Autodesk Fusion 360 part; units mm, degrees
note: some values were not read from the file. Set by a fixed rule: the direction of a hole.
(part 8 of 10)
  arc A350 (11.303, 28.321) -> (11.049, 28.575) centre (11.049, 28.321) ccw
  arc A351 (9.017, 28.321) -> (9.271, 28.575) centre (9.271, 28.321) cw
  line L6255 (11.049, 22.225) -> (9.271, 22.225)
  line L6256 (9.017, 22.479) -> (9.017, 22.86)
  line L6257 (9.144, 22.987) -> (9.017, 22.86)
  line L6258 (11.303, 22.479) -> (11.303, 22.86)
  line L6259 (11.176, 22.987) -> (11.303, 22.86)
  line L6260 (9.144, 27.813) -> (9.017, 27.94)
  line L6261 (9.144, 27.813) -> (9.144, 22.987)
  line L6262 (11.176, 27.813) -> (11.303, 27.94)
  line L6263 (11.176, 27.813) -> (11.176, 22.987)
  line L6264 (9.017, 28.321) -> (9.017, 27.94)
  line L6265 (11.303, 28.321) -> (11.303, 27.94)
  line L6266 (11.049, 28.575) -> (9.271, 28.575)
  line L6267 (9.8552, 28.575) -> (10.4648, 28.575)
  line L6268 (10.4648, 29.4386) -> (9.8552, 29.4386)
  line L6269 (9.8552, 29.4386) -> (9.8552, 28.575)
  line L6270 (10.4648, 28.575) -> (10.4648, 29.4386)
  line L6271 (9.8552, 22.225) -> (9.8552, 21.3614)
  line L6272 (9.8552, 21.3614) -> (10.4648, 21.3614)
  line L6273 (10.4648, 21.3614) -> (10.4648, 22.225)
  line L6274 (10.4648, 22.225) -> (9.8552, 22.225)
  arc A352 (21.971, 22.225) -> (21.717, 22.479) centre (21.971, 22.479) cw
  arc A353 (23.749, 22.225) -> (24.003, 22.479) centre (23.749, 22.479) ccw
  arc A354 (24.003, 28.321) -> (23.749, 28.575) centre (23.749, 28.321) ccw
  arc A355 (21.717, 28.321) -> (21.971, 28.575) centre (21.971, 28.321) cw
  line L6275 (23.749, 22.225) -> (21.971, 22.225)
  line L6276 (21.717, 22.479) -> (21.717, 22.86)
  line L6277 (21.844, 22.987) -> (21.717, 22.86)
  line L6278 (24.003, 22.479) -> (24.003, 22.86)
  line L6279 (23.876, 22.987) -> (24.003, 22.86)
  line L6280 (21.844, 27.813) -> (21.717, 27.94)
  line L6281 (21.844, 27.813) -> (21.844, 22.987)
  line L6282 (23.876, 27.813) -> (24.003, 27.94)
  line L6283 (23.876, 27.813) -> (23.876, 22.987)
  line L6284 (21.717, 28.321) -> (21.717, 27.94)
  line L6285 (24.003, 28.321) -> (24.003, 27.94)
  line L6286 (23.749, 28.575) -> (21.971, 28.575)
  line L6287 (22.5552, 28.575) -> (23.1648, 28.575)
  line L6288 (22.5552, 29.4386) -> (22.5552, 28.575)
  line L6289 (23.1648, 29.4386) -> (22.5552, 29.4386)
  line L6290 (23.1648, 28.575) -> (23.1648, 29.4386)
  line L6291 (22.5552, 21.3614) -> (23.1648, 21.3614)
  line L6292 (23.1648, 22.225) -> (22.5552, 22.225)
  line L6293 (23.1648, 21.3614) -> (23.1648, 22.225)
  line L6294 (22.5552, 22.225) -> (22.5552, 21.3614)
  arc A356 (34.671, 22.225) -> (34.417, 22.479) centre (34.671, 22.479) cw
  arc A357 (36.449, 22.225) -> (36.703, 22.479) centre (36.449, 22.479) ccw
  arc A358 (36.703, 28.321) -> (36.449, 28.575) centre (36.449, 28.321) ccw
  arc A359 (34.417, 28.321) -> (34.671, 28.575) centre (34.671, 28.321) cw
  line L6295 (36.449, 22.225) -> (34.671, 22.225)
  line L6296 (34.417, 22.479) -> (34.417, 22.86)
  line L6297 (34.544, 22.987) -> (34.417, 22.86)
  line L6298 (36.703, 22.479) -> (36.703, 22.86)
  line L6299 (36.576, 22.987) -> (36.703, 22.86)
  line L6300 (34.544, 27.813) -> (34.417, 27.94)
  line L6301 (34.544, 27.813) -> (34.544, 22.987)
  line L6302 (36.576, 27.813) -> (36.703, 27.94)
  line L6303 (36.576, 27.813) -> (36.576, 22.987)
  line L6304 (34.417, 28.321) -> (34.417, 27.94)
  line L6305 (36.703, 28.321) -> (36.703, 27.94)
  line L6306 (36.449, 28.575) -> (34.671, 28.575)
  line L6307 (35.8648, 28.575) -> (35.8648, 29.4386)
  line L6308 (35.2552, 29.4386) -> (35.2552, 28.575)
  line L6309 (35.8648, 29.4386) -> (35.2552, 29.4386)
  line L6310 (35.2552, 28.575) -> (35.8648, 28.575)
  line L6311 (35.8648, 22.225) -> (35.2552, 22.225)
  line L6312 (35.2552, 21.3614) -> (35.8648, 21.3614)
  line L6313 (35.8648, 21.3614) -> (35.8648, 22.225)
  line L6314 (35.2552, 22.225) -> (35.2552, 21.3614)
  arc A360 (47.371, 22.225) -> (47.117, 22.479) centre (47.371, 22.479) cw
  arc A361 (49.149, 22.225) -> (49.403, 22.479) centre (49.149, 22.479) ccw
  arc A362 (49.403, 28.321) -> (49.149, 28.575) centre (49.149, 28.321) ccw
  arc A363 (47.117, 28.321) -> (47.371, 28.575) centre (47.371, 28.321) cw
  line L6315 (49.149, 22.225) -> (47.371, 22.225)
  line L6316 (47.117, 22.479) -> (47.117, 22.86)
  line L6317 (47.244, 22.987) -> (47.117, 22.86)
  line L6318 (49.403, 22.479) -> (49.403, 22.86)
  line L6319 (49.276, 22.987) -> (49.403, 22.86)
  line L6320 (47.244, 27.813) -> (47.117, 27.94)
  line L6321 (47.244, 27.813) -> (47.244, 22.987)
  line L6322 (49.276, 27.813) -> (49.403, 27.94)
  line L6323 (49.276, 27.813) -> (49.276, 22.987)
  line L6324 (47.117, 28.321) -> (47.117, 27.94)
  line L6325 (49.403, 28.321) -> (49.403, 27.94)
  line L6326 (49.149, 28.575) -> (47.371, 28.575)
  line L6327 (47.9552, 28.575) -> (48.5648, 28.575)
  line L6328 (48.5648, 28.575) -> (48.5648, 29.4386)
  line L6329 (48.5648, 29.4386) -> (47.9552, 29.4386)
  line L6330 (47.9552, 29.4386) -> (47.9552, 28.575)
  line L6331 (47.9552, 21.3614) -> (48.5648, 21.3614)
  line L6332 (48.5648, 21.3614) -> (48.5648, 22.225)
  line L6333 (47.9552, 22.225) -> (47.9552, 21.3614)
  line L6334 (48.5648, 22.225) -> (47.9552, 22.225)
  arc A364 (52.451, 22.225) -> (52.197, 22.479) centre (52.451, 22.479) cw
  arc A365 (54.229, 22.225) -> (54.483, 22.479) centre (54.229, 22.479) ccw
  arc A366 (54.483, 28.321) -> (54.229, 28.575) centre (54.229, 28.321) ccw
  arc A367 (52.197, 28.321) -> (52.451, 28.575) centre (52.451, 28.321) cw
  line L6335 (54.229, 22.225) -> (52.451, 22.225)
  line L6336 (52.197, 22.479) -> (52.197, 22.86)
  line L6337 (52.324, 22.987) -> (52.197, 22.86)
  line L6338 (54.483, 22.479) -> (54.483, 22.86)
  line L6339 (54.356, 22.987) -> (54.483, 22.86)
  line L6340 (52.324, 27.813) -> (52.197, 27.94)
  line L6341 (52.324, 27.813) -> (52.324, 22.987)
  line L6342 (54.356, 27.813) -> (54.483, 27.94)
  line L6343 (54.356, 27.813) -> (54.356, 22.987)
  line L6344 (52.197, 28.321) -> (52.197, 27.94)
  line L6345 (54.483, 28.321) -> (54.483, 27.94)
  line L6346 (54.229, 28.575) -> (52.451, 28.575)
  line L6347 (53.0352, 29.4386) -> (53.0352, 28.575)
  line L6348 (53.6448, 28.575) -> (53.6448, 29.4386)
  line L6349 (53.0352, 28.575) -> (53.6448, 28.575)
  line L6350 (53.6448, 29.4386) -> (53.0352, 29.4386)
  line L6351 (53.6448, 22.225) -> (53.0352, 22.225)
  line L6352 (53.0352, 22.225) -> (53.0352, 21.3614)
  line L6353 (53.6448, 21.3614) -> (53.6448, 22.225)
  line L6354 (53.0352, 21.3614) -> (53.6448, 21.3614)
  arc A368 (66.421, 22.225) -> (66.167, 22.479) centre (66.421, 22.479) cw
  arc A369 (68.199, 22.225) -> (68.453, 22.479) centre (68.199, 22.479) ccw
  arc A370 (68.453, 28.321) -> (68.199, 28.575) centre (68.199, 28.321) ccw
  arc A371 (66.167, 28.321) -> (66.421, 28.575) centre (66.421, 28.321) cw
  line L6355 (68.199, 22.225) -> (66.421, 22.225)
  line L6356 (66.167, 22.479) -> (66.167, 22.86)
  line L6357 (66.294, 22.987) -> (66.167, 22.86)
  line L6358 (68.453, 22.479) -> (68.453, 22.86)
  line L6359 (68.326, 22.987) -> (68.453, 22.86)
  line L6360 (66.294, 27.813) -> (66.167, 27.94)
  line L6361 (66.294, 27.813) -> (66.294, 22.987)
  line L6362 (68.326, 27.813) -> (68.453, 27.94)
  line L6363 (68.326, 27.813) -> (68.326, 22.987)
  line L6364 (66.167, 28.321) -> (66.167, 27.94)
  line L6365 (68.453, 28.321) -> (68.453, 27.94)
  line L6366 (68.199, 28.575) -> (66.421, 28.575)
  line L6367 (67.0052, 29.4386) -> (67.0052, 28.575)
  line L6368 (67.6148, 28.575) -> (67.6148, 29.4386)
  line L6369 (67.0052, 28.575) -> (67.6148, 28.575)
  line L6370 (67.6148, 29.4386) -> (67.0052, 29.4386)
  line L6371 (67.0052, 22.225) -> (67.0052, 21.3614)
  line L6372 (67.0052, 21.3614) -> (67.6148, 21.3614)
  line L6373 (67.6148, 22.225) -> (67.0052, 22.225)
  line L6374 (67.6148, 21.3614) -> (67.6148, 22.225)
  arc A372 (77.851, 22.225) -> (77.597, 22.479) centre (77.851, 22.479) cw
  arc A373 (79.629, 22.225) -> (79.883, 22.479) centre (79.629, 22.479) ccw
  arc A374 (79.883, 28.321) -> (79.629, 28.575) centre (79.629, 28.321) ccw
  arc A375 (77.597, 28.321) -> (77.851, 28.575) centre (77.851, 28.321) cw
  line L6375 (79.629, 22.225) -> (77.851, 22.225)
  line L6376 (77.597, 22.479) -> (77.597, 22.86)
  line L6377 (77.724, 22.987) -> (77.597, 22.86)
  line L6378 (79.883, 22.479) -> (79.883, 22.86)
  line L6379 (79.756, 22.987) -> (79.883, 22.86)
  line L6380 (77.724, 27.813) -> (77.597, 27.94)
  line L6381 (77.724, 27.813) -> (77.724, 22.987)
  line L6382 (79.756, 27.813) -> (79.883, 27.94)
  line L6383 (79.756, 27.813) -> (79.756, 22.987)
  line L6384 (77.597, 28.321) -> (77.597, 27.94)
  line L6385 (79.883, 28.321) -> (79.883, 27.94)
  line L6386 (79.629, 28.575) -> (77.851, 28.575)
  line L6387 (79.0448, 29.4386) -> (78.4352, 29.4386)
  line L6388 (78.4352, 28.575) -> (79.0448, 28.575)
  line L6389 (79.0448, 28.575) -> (79.0448, 29.4386)
  line L6390 (78.4352, 29.4386) -> (78.4352, 28.575)
  line L6391 (79.0448, 21.3614) -> (79.0448, 22.225)
  line L6392 (78.4352, 21.3614) -> (79.0448, 21.3614)
  line L6393 (79.0448, 22.225) -> (78.4352, 22.225)
  line L6394 (78.4352, 22.225) -> (78.4352, 21.3614)
  arc A376 (89.281, 22.225) -> (89.027, 22.479) centre (89.281, 22.479) cw
  arc A377 (91.059, 22.225) -> (91.313, 22.479) centre (91.059, 22.479) ccw
  arc A378 (91.313, 28.321) -> (91.059, 28.575) centre (91.059, 28.321) ccw
  arc A379 (89.027, 28.321) -> (89.281, 28.575) centre (89.281, 28.321) cw
  line L6395 (91.059, 22.225) -> (89.281, 22.225)
  line L6396 (89.027, 22.479) -> (89.027, 22.86)
  line L6397 (89.154, 22.987) -> (89.027, 22.86)
  line L6398 (91.313, 22.479) -> (91.313, 22.86)
  line L6399 (91.186, 22.987) -> (91.313, 22.86)
  line L6400 (89.154, 27.813) -> (89.027, 27.94)
  line L6401 (89.154, 27.813) -> (89.154, 22.987)
  line L6402 (91.186, 27.813) -> (91.313, 27.94)
  line L6403 (91.186, 27.813) -> (91.186, 22.987)
  line L6404 (89.027, 28.321) -> (89.027, 27.94)
  line L6405 (91.313, 28.321) -> (91.313, 27.94)
  line L6406 (91.059, 28.575) -> (89.281, 28.575)
  line L6407 (89.8652, 29.4386) -> (89.8652, 28.575)
  line L6408 (90.4748, 29.4386) -> (89.8652, 29.4386)
  line L6409 (90.4748, 28.575) -> (90.4748, 29.4386)
  line L6410 (89.8652, 28.575) -> (90.4748, 28.575)
  line L6411 (90.4748, 21.3614) -> (90.4748, 22.225)
  line L6412 (90.4748, 22.225) -> (89.8652, 22.225)
  line L6413 (89.8652, 21.3614) -> (90.4748, 21.3614)
  line L6414 (89.8652, 22.225) -> (89.8652, 21.3614)
  arc A380 (36.9326, 76.3477) -> (37.2918, 76.3477) centre (37.1122, 76.1681) cw
  arc A381 (35.6753, 75.0905) -> (35.6753, 74.7312) centre (35.8549, 74.9109) ccw
  arc A382 (39.8062, 70.6003) -> (40.1655, 70.6003) centre (39.9859, 70.7799) ccw
  arc A383 (41.4227, 72.2168) -> (41.4227, 71.8576) centre (41.2431, 72.0372) cw
  line L6415 (35.6753, 75.0905) -> (36.9326, 76.3477)
  line L6416 (37.2918, 76.3477) -> (37.5612, 76.0783)
  line L6417 (37.5612, 75.8987) -> (37.5612, 76.0783)
  line L6418 (35.6753, 74.7312) -> (35.9447, 74.4618)
  line L6419 (36.1243, 74.4618) -> (35.9447, 74.4618)
  line L6420 (40.9737, 72.4862) -> (41.1533, 72.4862)
  line L6421 (40.9737, 72.4862) -> (37.5612, 75.8987)
  line L6422 (39.5368, 71.0493) -> (39.5368, 70.8697)
  line L6423 (39.5368, 71.0493) -> (36.1243, 74.4618)
  line L6424 (41.4227, 72.2168) -> (41.1533, 72.4862)
  line L6425 (39.8062, 70.6003) -> (39.5368, 70.8697)
  line L6426 (40.1655, 70.6003) -> (41.4227, 71.8576)
  line L6427 (41.6203, 70.8338) -> (41.0096, 71.4445)
  line L6428 (41.1892, 70.4028) -> (41.6203, 70.8338)
  line L6429 (40.5786, 71.0134) -> (41.1892, 70.4028)
  line L6430 (41.0096, 71.4445) -> (40.5786, 71.0134)
  line L6431 (35.9088, 76.5453) -> (35.4778, 76.1142)
  line L6432 (36.0884, 75.5036) -> (36.5195, 75.9346)
  line L6433 (35.4778, 76.1142) -> (36.0884, 75.5036)
  line L6434 (36.5195, 75.9346) -> (35.9088, 76.5453)
  arc A384 (27.94, 75.311) -> (26.6999, 75.9492) centre (27.94, 76.835) cw
  arc A385 (29.1592, 75.9206) -> (27.94, 75.311) centre (27.94, 76.835) cw
  arc A386 (27.94, 78.359) -> (26.737, 77.7706) centre (27.94, 76.835) ccw
  arc A387 (29.143, 77.7706) -> (27.94, 78.359) centre (27.94, 76.835) ccw
  arc A388 (27.94, 74.803) -> (26.379, 75.5341) centre (27.94, 76.835) cw
  arc A389 (29.7329, 75.8788) -> (27.94, 74.803) centre (27.9399, 76.835) cw
  arc A390 (27.94, 78.867) -> (26.3888, 78.1476) centre (27.94, 76.835) ccw
  arc A391 (29.7043, 77.8432) -> (27.94, 78.867) centre (27.9401, 76.835) ccw
  arc A392 (6.731, 3.81) -> (0.889, 3.81) centre (3.81, 3.81) ccw
  arc A393 (0.889, 3.81) -> (6.731, 3.81) centre (3.81, 3.81) ccw
  arc A394 (5.31, 3.81) -> (2.31, 3.81) centre (3.81, 3.81) ccw
  arc A395 (2.31, 3.81) -> (5.31, 3.81) centre (3.81, 3.81) ccw
  arc A396 (99.441, 76.2) -> (93.599, 76.2) centre (96.52, 76.2) ccw
  arc A397 (93.599, 76.2) -> (99.441, 76.2) centre (96.52, 76.2) ccw
  arc A398 (95.02, 76.2) -> (98.02, 76.2) centre (96.52, 76.2) ccw
  arc A399 (98.02, 76.2) -> (95.02, 76.2) centre (96.52, 76.2) ccw
  arc A400 (6.731, 76.2) -> (0.889, 76.2) centre (3.81, 76.2) ccw
  arc A401 (0.889, 76.2) -> (6.731, 76.2) centre (3.81, 76.2) ccw
  arc A402 (2.31, 76.2) -> (5.31, 76.2) centre (3.81, 76.2) ccw
  arc A403 (5.31, 76.2) -> (2.31, 76.2) centre (3.81, 76.2) ccw
  arc A404 (99.441, 3.81) -> (93.599, 3.81) centre (96.52, 3.81) ccw
  arc A405 (93.599, 3.81) -> (99.441, 3.81) centre (96.52, 3.81) ccw
  arc A406 (98.02, 3.81) -> (95.02, 3.81) centre (96.52, 3.81) ccw
  arc A407 (95.02, 3.81) -> (98.02, 3.81) centre (96.52, 3.81) ccw
sketch "Skizze2" plane through (0, 0, 0) normal (1, 0, 0) x (0, 1, 0)
  line L0 (0, 80) -> (100.2, 80)
  line L1 (100.2, 80) -> (100.2, -0.2)
  line L2 (100.2, -0.2) -> (0, -0.2)
  line L3 (0, -0.2) -> (0, 80)
  line L4 (101.8, -1.8) -> (-1.6, -1.8)
  line L5 (-1.6, -1.8) -> (-1.6, 81.6)
  line L6 (-1.6, 81.6) -> (101.8, 81.6)
  line L7 (101.8, 81.6) -> (101.8, -1.8)
  line L8 (0, 80) -> (8, 80)
  line L9 (8, 78.8) -> (8, 73.1314)
  line L10 (6.8686, 72) -> (1.2, 72)
  line L11 (0, 72) -> (0, 80)
  line L12 (100.2, 80) -> (92.2, 80)
  line L13 (92.2, 78.8) -> (92.2, 73.1314)
  line L14 (93.3314, 72) -> (99, 72)
  line L15 (100.2, 72) -> (100.2, 80)
  line L16 (100.2, -0.2) -> (92.2, -0.2)
  line L17 (92.2, 1) -> (92.2, 6.9305)
  line L18 (94.2415, 7.8) -> (99, 7.8)
  line L19 (100.2, 7.8) -> (100.2, -0.2)
  line L20 (100.2, 50) -> (100.2, 36.72)
  line L21 (0, 36.72) -> (0, 50)
  line L22 (7.4343, 71.4343) -> (28.8686, 50)
  line L23 (8.5657, 72.5657) -> (30.5657, 50.5657)
  line L24 (91.6343, 72.5657) -> (69.6343, 50.5657)
  line L25 (92.7657, 71.4343) -> (71.3314, 50)
  line L26 (7.4343, 71.4343) -> (6.8686, 72)
  line L27 (8.5657, 72.5657) -> (8, 73.1314)
  line L28 (30.5657, 50.5657) -> (31.1314, 50)
  line L29 (1.2, 50) -> (28.8686, 50)
  line L30 (91.6343, 72.5657) -> (92.2, 73.1314)
  line L31 (92.7657, 71.4343) -> (93.3314, 72)
  line L32 (69.6343, 50.5657) -> (69.0686, 50)
  line L33 (71.3314, 50) -> (99, 50)
  line L34 (0, -0.2) -> (8, -0.2)
  line L35 (8, 1) -> (8, 6.9353)
  line L36 (5.8929, 7.8) -> (1.2, 7.8)
  line L37 (0, 7.8) -> (0, -0.2)
  line L38 (15.2532, 36.72) -> (15.2532, 21.72)
  line L39 (13.6532, 21.72) -> (13.6532, 36.72)
  line L40 (13.6532, 21.72) -> (13.6532, 11.72)
  line L41 (15.2532, 21.72) -> (15.2532, 11.72)
  line L42 (13.6532, 36.72) -> (1.2, 36.72)
  line L43 (85.1532, 21.72) -> (85.1532, 36.72)
  line L44 (86.7532, 36.72) -> (86.7532, 21.72)
  line L45 (85.1532, 21.72) -> (85.1532, 11.72)
  line L46 (86.7532, 21.72) -> (86.7532, 11.72)
  line L47 (99, 36.72) -> (86.7532, 36.72)
  line L48 (85.1532, 36.72) -> (15.2532, 36.72)
  line L49 (15.2532, 11.72) -> (85.1532, 11.72)
  line L50 (84.7118, 10.12) -> (15.7604, 10.12)
  line L51 (13.6532, 10.9848) -> (13.6532, 11.72)
  line L52 (86.7532, 11.72) -> (86.7532, 10.9896)
  line L53 (8.3037, 7.0599) -> (13.957, 9.3799)
  line L54 (7.6963, 8.5401) -> (13.3495, 10.8601)
  line L55 (13.957, 9.3799) -> (15.7604, 10.12)
  line L56 (13.3495, 10.8601) -> (13.6532, 10.9848)
  line L57 (8.3037, 7.0599) -> (8, 6.9353)
  line L58 (7.6963, 8.5401) -> (5.8929, 7.8)
  line L59 (86.4397, 9.384) -> (91.8865, 7.064)
  line L60 (87.0667, 10.856) -> (92.5135, 8.536)
  line L61 (92.5135, 8.536) -> (94.2415, 7.8)
  line L62 (91.8865, 7.064) -> (92.2, 6.9305)
  line L63 (86.4397, 9.384) -> (84.7118, 10.12)
  line L64 (87.0667, 10.856) -> (86.7532, 10.9896)
  line L65 (92.2, 1) -> (8, 1)
  line L66 (1.2, 7.8) -> (1.2, 36.72)
  line L67 (1.2, 50) -> (1.2, 72)
  line L68 (99, 72) -> (99, 50)
  line L69 (99, 36.72) -> (99, 7.8)
  line L70 (53.4782, 50) -> (53.4782, 67.3952)
  line L71 (53.4782, 68.9952) -> (47.2819, 68.9952)
  line L72 (45, 50) -> (47.2819, 50)
  line L73 (53.4782, 50) -> (55, 50)
  line L74 (31.1314, 50) -> (47.2819, 50)
  line L75 (53.4782, 50) -> (69.0686, 50)
  line L76 (45.033, 78.8) -> (45.033, 69)
  line L77 (45.033, 69) -> (47.2819, 68.9952)
  line L78 (56.3866, 78.8) -> (56.3866, 68.9952)
  line L79 (56.3866, 68.9952) -> (53.4782, 68.9952)
  line L80 (43.433, 78.8) -> (43.433, 67.4034)
  line L81 (43.433, 67.4034) -> (47.2785, 67.3952)
  line L82 (57.9866, 78.8) -> (57.9866, 67.3952)
  line L83 (57.9866, 67.3952) -> (53.4782, 67.3952)
  line L84 (8, 78.8) -> (43.433, 78.8)
  line L85 (45.033, 78.8) -> (56.3866, 78.8)
  line L86 (57.9866, 78.8) -> (92.2, 78.8)
  line L87 (47.2785, 67.3952) -> (47.2819, 50)
  line L88 (1.2, 47.7704) -> (99, 47.7704)
  line L89 (99, 47.7704) -> (99, 39)
  line L90 (99, 39) -> (1.2, 39)
  line L91 (1.2, 39) -> (1.2, 47.7704)
  dimension "d1" = 100.2
  dimension "d2" = 80.2
  dimension "d5" = -1.6
  dimension "d8" = 8
  dimension "d9" = 8
  dimension "d10" = 8
  dimension "d11" = 8
  dimension "d12" = 8
  dimension "d13" = 8
  dimension "d21" = 8
  dimension "d22" = 8
  dimension "d23" = 1.6
  dimension "d24" = 15
  dimension "d25" = 10
  dimension "d26" = 10
  dimension "d27" = 1.6
  dimension "d28" = 15
  dimension "d29" = 10
  dimension "d30" = 10
  dimension "d37" = 1.6
  dimension "d38" = -1.6
  constraint horizontal L0
  constraint vertical L1
  constraint horizontal L2
  constraint vertical L3
  constraint horizontal L8
  constraint vertical L9
  constraint horizontal L10
  constraint vertical L11
  constraint horizontal L12
  constraint vertical L13
  constraint horizontal L14
  constraint vertical L15
  constraint horizontal L16
  constraint vertical L17
  constraint horizontal L18
  constraint vertical L19
  constraint horizontal L29
  constraint vertical L20
  constraint horizontal L47
  constraint vertical L21
  constraint coincident L1 L20.end
  constraint coincident L3 L21.end
  constraint horizontal L72
  constraint coincident L72.start L29
  constraint parallel L23 L27
  constraint coincident L28.end L29
  constraint parallel L23 L28
  constraint collinear L29 L74
  constraint parallel L24 L30
  constraint parallel L25 L31
  constraint parallel L24 L32
  constraint collinear L33 L74
  constraint horizontal L34
  constraint vertical L35
  constraint horizontal L36
  constraint vertical L37
  constraint vertical L38
  constraint vertical L39
  constraint coincident L39.end L47
  constraint collinear L42 L47
  constraint vertical L44
  constraint vertical L43
  constraint collinear L47 L48
  constraint horizontal L49
  constraint horizontal L50
  constraint vertical L51
  constraint perpendicular L50 L52
  constraint parallel L53 L55
  constraint parallel L54 L56
  constraint parallel L53 L57
  constraint parallel L54 L58
  constraint parallel L60 L61
  constraint parallel L59 L62
  constraint parallel L59 L63
  constraint parallel L60 L64
  constraint collinear L66 L67
  constraint collinear L68 L69
  constraint vertical L70
  constraint horizontal L71
  constraint collinear L72 L73
  constraint collinear L74 L75
  constraint coincident L76.start L84
  constraint perpendicular L76 L84
  constraint coincident L78.start L84
  constraint perpendicular L78 L84
  constraint perpendicular L70 L79
  constraint collinear L84 L85
  constraint collinear L85 L86
  constraint horizontal L88
  constraint vertical L89
  constraint horizontal L90
  constraint vertical L91
  measures "d1" distance of L0.start L0.end
  measures "d2" distance of L0.start L2.end
  measures "d8" distance of L0.start L8.end
  measures "d9" distance of L0.start L11.start
  measures "d10" distance of L0.end L12.end
  measures "d11" distance of L0.end L15.start
  measures "d12" distance of L1.end L16.end
  measures "d13" distance of L1.end L19.start
  measures "d21" distance of L2.end L34.end
  measures "d22" distance of L2.end L37.start
  measures "d23" distance of L39.end L38.start
  measures "d24" distance of L39.end L39.start
  measures "d25" distance of L39.start L40.end
  measures "d26" distance of L38.end L41.end
  measures "d27" distance of L44.start L43.end
  measures "d28" distance of L43.end L43.start
  measures "d29" distance of L43.start L45.end
  measures "d30" distance of L44.end L46.end